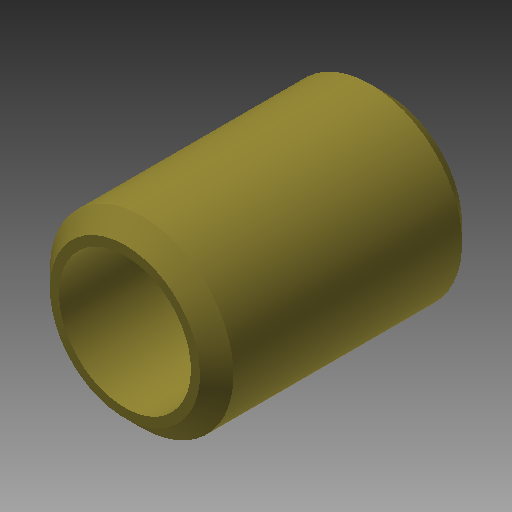
# Autodesk Inventor part: D-8597
Saved by Autodesk Inventor 2018 (Build 220112000, 112)
## iProperties
Category: PARTsolutions
Company: BIMBA
Created: 2019-01-18
Part Number: D-8597
Material: Generic
Catalog Web Link: www.cadenas.de
Description: Bushing-Original Line - Standard Air Cylinders
Vendor: BIMBA
Document SubType Name: Modeling
Designer: psadmin
Manufacturer: BIMBA
Mass: 0.0885073 g
Surface Area: 2.4981 cm^2
Volume: 0.0885073 cm^3
Density: 1 g/cm^3
Appearance: PSOLRGB-181-165-66
PSOL_IDENT_0: {$CADENAS_DATA\23d-libs\bimba\bimba\bimba_imperial\bimba_full_line\original_line_cylinders\standard_
PSOL_IDENT_1: air_cylinders\bushing.prj},153 {VTYP=3D},{NB=D-8597},{LINA=D-8597},{NN=Bushing},{DATE=21.03.2018 14:
PSOL_IDENT_2: 31:21},{GEOMDATE=10.09.2012 00:00:00},{VERSION=},{LINEID=20},{WBVAR=},{WBNUMERIC=}  {NB=D-8597},{LIN
PSOL_IDENT_3: A=D-8597},{KT=DUMMY},{PN=D-8597},{ID=0.1570},{OD=0.2185},{L=0.3120},{C=0.0200}
NN: Bushing
NT: Original Line - Standard Air Cylinders
NB: D-8597
NBSYN: $PN.
LINA: D-8597
PN: D-8597
ID: 0.157
OD: 0.2185
L: 0.312
C: 0.02
SUPPLIER: BIMBA
ARTICLENO: D-8597
BOMINFO: D-8597
CREATOR: CADENAS GmbH
Title: D-8597
Author: Cadenas PARTsolutions
Comments: Original Line - Standard Air Cylinders
Autodesk Inventor part; units mm, degrees
sketch "Sketch_1" plane through (0, 0, 0) normal (1, 0, 0) x (0, 1, 0)
  line L0 (0, -3.9624) -> (0, 3.9624)
  line L1 (1.9939, 3.9624) -> (1.9939, -3.9624)
  line L2 (1.9939, -3.9624) -> (2.267, -3.9624)
  line L3 (2.267, -3.9624) -> (2.775, -3.4544)
  line L4 (2.775, -3.4544) -> (2.775, 3.4544)
  line L5 (2.775, 3.4544) -> (2.267, 3.9624)
  line L6 (2.267, 3.9624) -> (1.9939, 3.9624)
  constraints: 14 end point
revolve "Revolution1" add sketch "Sketch_1" angle 360 about axis through (0, 0, -3.9624) along (0, 0, -1)
ref_plane "bushing_XY" through (0, 0, 0) normal (0, 0, 1) x (1, 0, 0)
ref_plane "bushing_YZ" through (0, 0, 0) normal (1, 0, 0) x (0, 1, 0)
ref_plane "bushing_ZX" through (0, 0, 0) normal (0, 1, 0) x (0, 0, 1)
ref_plane "id1_XY" through (-1.9939, 0, 0) normal (0, 0, 1) x (1, 0, 0)
ref_plane "id1_YZ" through (-1.9939, 0, 0) normal (1, 0, 0) x (0, 1, 0)
ref_plane "id1_ZX" through (-1.9939, 0, 0) normal (0, 1, 0) x (0, 0, 1)
ref_plane "id2_XY" through (1.9939, 0, 0) normal (0, 0, 1) x (1, 0, 0)
ref_plane "id2_YZ" through (1.9939, 0, 0) normal (1, 0, 0) x (0, 1, 0)
ref_plane "id2_ZX" through (1.9939, 0, 0) normal (0, 1, 0) x (0, 0, 1)
ref_plane "id3_XY" through (0, 0, -3.9624) normal (0, 0, -1) x (0, 1, 0)
ref_plane "id3_YZ" through (0, 0, -3.9624) normal (0, 1, 0) x (1, 0, 0)
ref_plane "id3_ZX" through (0, 0, -3.9624) normal (1, 0, 0) x (0, 0, -1)
ref_plane "id4_XY" through (0, 0, 3.9624) normal (0, 0, 1) x (0, 1, 0)
ref_plane "id4_YZ" through (0, 0, 3.9624) normal (0, 1, 0) x (-1, 0, 0)
ref_plane "id4_ZX" through (0, 0, 3.9624) normal (-1, 0, 0) x (0, 0, 1)
body "Solid1"
